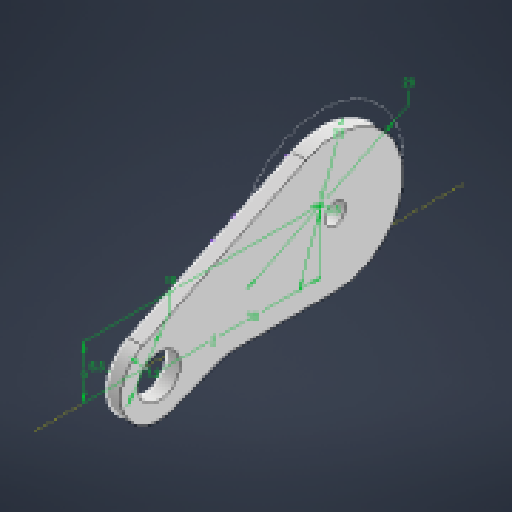
# Autodesk Inventor part: Gear_Cover
Saved by Autodesk Inventor 2024.2 (Build 282272000, 272)
## iProperties
Created: 2024-02-26
Part Number: Gear_Cover
Material: 一般
Document SubType Name: Modeling
Designer: Hanaoka
Density: 1 g/cm^3
Appearance: 既定
Author: Hanaoka
Autodesk Inventor part; units mm, degrees
ref_plane "YZ Plane" through (0, 0, 0) normal (1, 0, 0) x (0, 1, 0)
ref_plane "XZ Plane" through (0, 0, 0) normal (0, 1, 0) x (-1, 0, 0)
ref_plane "XY Plane" through (0, 0, 0) normal (0, 0, 1) x (1, 0, 0)
sketch "スケッチ1" plane through (0, 0, 0) normal (1, 0, 0) x (0, 1, 0)
  circle A0 centre (0, 0) radius 3.6
  arc A1 (5.8479, 2.8377) -> (-6.0569, -2.3587) centre (0, 0) ccw
  line L0 (-6.0569, -2.3587) -> (-2.6363, -11.1423)
  line L1 (-2.5, -11.8681) -> (-2.5, -30)
  line L2 (0, -54.5111) -> (0, 19.0665) construction
  circle A2 centre (0, 0) radius 5 construction
  line L3 (4.8885, 1.0499) -> (11.4443, -29.4751) construction
  line L4 (-4.6592, -1.8144) -> (6.6704, -30.9072) construction
  circle A3 centre (9, -30) radius 14 construction
  circle A4 centre (9, -30) radius 2.5 construction
  circle A5 centre (9, -30) radius 11.5
  arc A6 (-2.5, -11.8681) -> (-2.6363, -11.1423) centre (-4.5, -11.8681) ccw
  line L5 (5.8479, 2.8377) -> (19.3462, -24.9795)
  circle A7 centre (9, -30) radius 1.75
  point P0 (-2.5, -11.4924)
  point P1 (19.0229, -24.3617)
  point P2 (12.8525, -11.5974)
  point P3 (14.5988, -15.1961)
  dimension "d0" = 7.2
  dimension "d1" = 6.5
  dimension "d3" = 10
  dimension "d4" = 28
  dimension "d5" = 5
  dimension "d6" = 23
  dimension "d10" = 30
  dimension "d11" = 9
  dimension "d12" = 3.5
  dimension "d13" = 2
  constraints: 11 point on circle, 10 end point, 10 tangent, 8 centre point, 6 coincident, 4 point on line, 1 parallel, 1 vertical
  measures "d0" diameter of A0
  measures "d1" radius of A1
  measures "d3" diameter of A2
  measures "d4" diameter of A3
  measures "d5" diameter of A4
  measures "d6" diameter of A5
  measures "d10" vertical distance of A3.centre point (0, 0)
  measures "d11" horizontal distance of A3.centre point (0, 0)
  measures "d12" diameter of A7
  measures "d13" radius of A6
extrude "押し出し1" add sketch "スケッチ1" along normal blind 2.5
